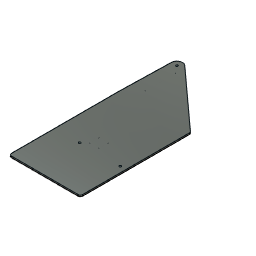
BoltPlade v1 (Autodesk Fusion 360 design; units mm, degrees)
Autodesk Fusion 360 part; units mm, degrees
note: some values were not read from the file. Set by a fixed rule: which sketch regions a step uses.
sketch "Sketch1" plane through (0, 0, 0) normal (0, 0, 1) x (1, 0, 0)
  line L0 (0, 0) -> (300, 0)
  line L1 (300, 0) -> (300, 335)
  line L2 (300, 335) -> (0, 335)
  line L3 (0, 335) -> (0, 0)
  line L4 (0, 0) -> (100, 0)
  line L5 (100, 0) -> (100, 60)
  line L6 (100, 60) -> (0, 60)
  line L7 (0, 60) -> (0, 0)
  line L8 (300, 0) -> (280, 0)
  line L9 (280, 0) -> (280, 60)
  line L10 (280, 60) -> (300, 60)
  line L11 (300, 60) -> (300, 0)
  line L12 (0, 335) -> (300, 335)
  line L13 (300, 335) -> (300, 670)
  line L14 (300, 670) -> (0, 670)
  line L15 (0, 670) -> (0, 335)
  line L16 (0, 670) -> (20, 670)
  line L17 (20, 670) -> (20, 570)
  line L18 (20, 570) -> (0, 570)
  line L19 (0, 570) -> (0, 670)
  circle A0 centre (20, 570) radius 4.5
  circle A1 centre (280, 60) radius 4.5
  circle A2 centre (100, 60) radius 4.5
  line L20 (20, 570) -> (20, 530)
  line L21 (20, 530) -> (74, 530)
  line L22 (74, 530) -> (74, 410)
  line L23 (74, 410) -> (20, 410)
  line L24 (20, 410) -> (20, 530)
  line L25 (0, 335) -> (124, 335)
  line L26 (124, 335) -> (124, 121.3118)
  line L27 (124, 121.3118) -> (0, 121.3118)
  line L28 (0, 121.3118) -> (0, 335)
  circle A3 centre (124, 121.3118) radius 0.5
  line L29 (124, 121.3118) -> (164, 121.3118)
  line L30 (164, 121.3118) -> (164, 81.3118)
  line L31 (164, 81.3118) -> (124, 81.3118)
  line L32 (124, 81.3118) -> (124, 121.3118)
  circle A4 centre (164, 121.3118) radius 0.5
  circle A5 centre (164, 81.3118) radius 0.5
  circle A6 centre (124, 81.3118) radius 0.5
  line L33 (47, 530) -> (47, 537.5)
  circle A7 centre (47, 537.5) radius 0.5
  line L34 (47, 410) -> (47, 402.5)
  circle A8 centre (47, 402.5) radius 0.5
  line L35 (0, 335) -> (295.006, 335)
  line L36 (295.006, 335) -> (295.006, -131.766)
  line L37 (295.006, -131.766) -> (0, -131.766)
  line L38 (0, -131.766) -> (0, 335)
  line L39 (-10, 345) -> (305.006, 345)
  line L40 (305.006, 340.5643) -> (305.006, -131.766)
  line L41 (295.006, -141.766) -> (0, -141.766)
  line L42 (-10, -131.766) -> (-10, 345)
  circle A9 centre (20, 570) radius 24.5
  circle A10 centre (100, 60) radius 24.5
  circle A11 centre (280, 60) radius 24.5
  line L43 (301.7178, 347.9772) -> (36.444, 588.1617)
  line L44 (-10, 345) -> (-4.4927, 570.5979)
  arc A12 (-10, -131.766) -> (0, -141.766) centre (0, -131.766) ccw
  arc A13 (295.006, -141.766) -> (305.006, -131.766) centre (295.006, -131.766) ccw
  arc A14 (305.006, 340.5643) -> (301.7178, 347.9772) centre (295.006, 340.5643) ccw
  dimension "d1" = 300
  dimension "d2" = 335
  dimension "d3" = 100
  dimension "d4" = 60
  dimension "d5" = 20
  dimension "d6" = 60
  dimension "d7" = 300
  dimension "d8" = 335
  dimension "d9" = 20
  dimension "d10" = 100
  dimension "d11" = 9
  dimension "d12" = 9
  dimension "d13" = 9
  dimension "d14" = 40
  dimension "d15" = 54
  dimension "d16" = 120
  dimension "d17" = 124
  dimension "d18" = 213.6882
  dimension "d19" = 1
  dimension "d20" = 40
  dimension "d21" = 40
  dimension "d22" = 1
  dimension "d23" = 1
  dimension "d24" = 1
  dimension "d25" = 7.5
  dimension "d26" = 1
  dimension "d27" = 7.5
  dimension "d28" = 1
  dimension "d29" = 295.006
  dimension "d30" = 466.766
  dimension "d32" = 20
  dimension "d33" = 20
  dimension "d34" = 20
  dimension "d35" = 10
  dimension "d36" = 10
  constraint horizontal L0
  constraint vertical L1
  constraint horizontal L2
  constraint vertical L3
  constraint coincident L0.start L3.end
  constraint horizontal L4
  constraint vertical L5
  constraint horizontal L6
  constraint vertical L7
  constraint horizontal L8
  constraint vertical L9
  constraint horizontal L10
  constraint vertical L11
  constraint horizontal L12
  constraint vertical L13
  constraint horizontal L14
  constraint vertical L15
  constraint horizontal L16
  constraint vertical L17
  constraint horizontal L18
  constraint vertical L19
  constraint coincident L17.end L18.start
  constraint coincident L9.end L10.start
  constraint coincident L5.end L6.start
  constraint perpendicular L18 L20
  constraint horizontal L21
  constraint vertical L22
  constraint horizontal L23
  constraint vertical L24
  constraint horizontal L25
  constraint vertical L26
  constraint horizontal L27
  constraint vertical L28
  constraint coincident L26.end L27.start
  constraint horizontal L29
  constraint vertical L30
  constraint horizontal L31
  constraint vertical L32
  constraint coincident L29.end L30.start
  constraint coincident L30.end L31.start
  constraint coincident L31.end L32.start
  constraint midpoint L21 L33.start
  constraint perpendicular L21 L33
  constraint coincident L33.end A7.centre
  constraint midpoint L23 L34.start
  constraint perpendicular L23 L34
  constraint coincident L34.end A8.centre
  constraint horizontal L35
  constraint vertical L36
  constraint horizontal L37
  constraint vertical L38
  constraint coincident A9 L43.end
  constraint tangent A9 L43
  constraint coincident A9 L44.end
  constraint tangent A9 L44
  constraint tangent L42 A12
  constraint tangent L41 A12
  constraint tangent L40 A13
  constraint tangent L41 A13
  constraint equal A12 A13
  constraint coincident L39.end L43
  constraint coincident L39.end L40
  constraint tangent L43 A14
  constraint tangent L40 A14
  measures "d1" distance of L0.start L0.end
  measures "d2" distance of L0.start L2.end
  measures "d3" distance of L0.start L4.end
  measures "d4" distance of L0.start L6.end
  measures "d5" distance of L0.end L8.end
  measures "d6" distance of L0.end L10.end
  measures "d7" distance of L2.end L1.end
  measures "d8" distance of L2.end L14.end
  measures "d9" distance of L14.end L16.end
  measures "d10" distance of L14.end L18.end
  measures "d11" diameter of A0
  measures "d12" diameter of A1
  measures "d13" diameter of A2
  measures "d14" distance of L17.end L20.end
  measures "d15" distance of L20.end L21.end
  measures "d16" distance of L20.end L23.end
  measures "d17" distance of L2.end L25.end
  measures "d18" distance of L2.end L27.end
  measures "d19" diameter of A3
  measures "d20" distance of L26.end L29.end
  measures "d21" distance of L26.end L31.end
  measures "d22" diameter of A4
  measures "d23" diameter of A5
  measures "d24" diameter of A6
  measures "d25" distance of L33.start L33.end
  measures "d26" diameter of A7
  measures "d27" distance of L34.start L34.end
  measures "d28" diameter of A8
  measures "d29" distance of L2.end L35.end
  measures "d30" distance of L2.end L37.end
  measures "d35" radius of A12
  measures "d36" radius of A14
extrude "Extrude1" add sketch "Sketch1" along normal blind 6 contours L0 L3 L4 L5 L6 L7 L38 A10 | L0 L1 L3 L7 L8 L11 L13 L15 L28 L36 L37 L38 L39 L40 L41 L42 A11 A12 A13 A14 | L0 L4 L8 L36 L37 L38 | L0 L2 L3 L5 L6 L9 L12 L26 L27 A3 L29 L30 L31 L32 A4 A5 A6 L35 L36 L38 A10 A11 | L0 L8 L9 L36 A11 | L5 L6 A2 A10 | L5 L6 A2 A10 | L2 L3 L12 L25 L26 L27 L28 A3 L35 L38 | L0 L1 L8 L11 L36 A11 | L9 L10 A1 L36 A11 | L9 L10 A1 L36 A11 | L2 L12 L13 L15 L25 L35 L39 | L1 L10 L11 L36 A11 | L1 L10 L36 A11 | L1 L2 L12 L36 A11 | L15 L39 A9 L44 | L13 L15 L39 A9 L43 | A3 L29 L30 L31 L32 A4 A5 A6 | L1 L11 A11 | L15 L19 A9 | L15 L18 A0 L20 A9 | L13 L39 L43 A14 | L15 L17 L18 L19 A0 A9 | L17 A0 L20 A9 | L21 L22 L23 L24
sketch "FaceSketch" plane through (0, 0, 6) normal (0, 0, 1) x (-1, 0, 0)
  circle A0 centre (-124, -81.3118) radius 0.5
  circle A1 centre (-164, -121.3118) radius 0.5
  circle A2 centre (-280, -60) radius 4.5
  circle A3 centre (-20, -570) radius 4.5
  circle A4 centre (-47, -402.5) radius 0.5
  circle A5 centre (-124, -121.3118) radius 0.5
  circle A6 centre (-47, -537.5) radius 0.5
  circle A7 centre (-100, -60) radius 4.5
  circle A8 centre (-164, -81.3118) radius 0.5
  arc A9 (-295.006, 141.766) -> (-305.006, 131.766) centre (-295.006, 131.766) ccw
  line L0 (-305.006, 131.766) -> (-305.006, -340.5643)
  arc A10 (-305.006, -340.5643) -> (-301.7178, -347.9772) centre (-295.006, -340.5643) ccw
  line L1 (-301.7178, -347.9772) -> (-36.444, -588.1617)
  arc A11 (-36.444, -588.1617) -> (4.4927, -570.5979) centre (-20, -570) ccw
  line L2 (4.4927, -570.5979) -> (10, -345)
  line L3 (10, -345) -> (10, 131.766)
  arc A12 (10, 131.766) -> (0, 141.766) centre (0, 131.766) ccw
  line L4 (0, 141.766) -> (-295.006, 141.766)
equation "d19 = d26"
equation "d22 = d19"
equation "d23 = d19"
equation "d24 = d19"
equation "d28 = d26"
